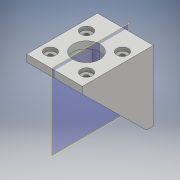
# Autodesk Inventor part: CarroXY-Motor
Saved by Autodesk Inventor 2017 (Build 210142000, 142)
## iProperties
Created: 2020-08-14
Part Number: CarroXY-Motor
Material: Generic
Document SubType Name: Modeling
Designer: ale
Density: 1 g/cm^3
Appearance: Default
Author: ale
Autodesk Inventor part; units mm, degrees
ref_plane "YZ Plane" through (0, 0, 0) normal (1, 0, 0) x (0, 1, 0)
ref_plane "XZ Plane" through (0, 0, 0) normal (0, 1, 0) x (-1, 0, 0)
ref_plane "XY Plane" through (0, 0, 0) normal (0, 0, 1) x (1, 0, 0)
sketch "Sketch1" plane through (0, 0, 0) normal (0, 0, 1) x (1, 0, 0)
  line L0 (-24, 27.5) -> (24, 27.5)
  line L1 (24, 27.5) -> (24, -27.5)
  line L2 (24, -27.5) -> (-24, -27.5)
  line L3 (-24, -27.5) -> (-24, 27.5)
  line L4 (-24, 27.5) -> (24, -27.5) construction
  line L5 (24, 27.5) -> (-24, -27.5) construction
  circle A0 centre (0, 0) radius 11.5
  line L6 (-15.5, 15.5) -> (15.5, -15.5) construction
  line L7 (15.5, 15.5) -> (-15.5, -15.5) construction
  circle A1 centre (-15.5, 15.5) radius 2
  circle A2 centre (15.5, 15.5) radius 2
  circle A3 centre (-15.5, -15.5) radius 2
  circle A4 centre (15.5, -15.5) radius 2
  dimension "d0" = 48
  dimension "d1" = 55
  dimension "d2" = 23
  dimension "d3" = 31
  dimension "d4" = 31
  dimension "d5" = 4
  dimension "d6" = 4
  dimension "d7" = 4
  dimension "d8" = 4
  constraints: 16 end point, 5 centre point, 5 coincident, 4 midpoint, 2 parallel, 1 horizontal, 1 perpendicular
  measures "d0" distance of L1.end L2.end
  measures "d1" distance of L0.end L1.end
  measures "d2" diameter of A0
  measures "d3" distance of L6.end L7.end
  measures "d4" distance of L7.start L6.end
  measures "d5" diameter of A1
  measures "d6" diameter of A2
  measures "d7" diameter of A3
  measures "d8" diameter of A4
extrude "Extrusion1" add sketch "Sketch1" along normal blind 6
sketch "Sketch2" plane through (0, 0, 6) normal (0, 0, 1) x (1, 0, 0)
  circle A0 centre (-15.5, 15.5) radius 2 projected
  circle A1 centre (15.5, 15.5) radius 2 projected
  circle A2 centre (15.5, -15.5) radius 2 projected
  circle A3 centre (-15.5, -15.5) radius 2 projected
  point P0 (0, 0)
  constraints: 4 coincident
hole "Hole1" at (-15.5, 15.5, 6) at (15.5, 15.5, 6) at (15.5, -15.5, 6) at (-15.5, -15.5, 6) direction (0, 0, -1) diameter 4 end through all counterbore diameter 10 counterbore depth 3
sketch "Sketch4" plane through (-24, 27.5, 0) normal (0, 1, 0) x (1, 0, 0)
  line L0 (0, 0) -> (0, -6) projected
  line L1 (0, -6) -> (48, -6)
  line L2 (48, -6) -> (48, 54)
  line L3 (48, 54) -> (0, 54)
  line L4 (0, 54) -> (0, -6)
  point P0 (24, 0)
  dimension "d20" = 60
  constraints: 8 end point, 2 parallel, 1 horizontal, 1 perpendicular
  measures "d20" distance of L2.end L1.end
extrude "Extrusion2" add sketch "Sketch4" along normal blind 6
sketch "Sketch5" plane through (-24, 27.5, 0) normal (0, -1, 0) x (1, 0, 0)
  arc A0 (7.75, -44) -> (12.25, -44) centre (10, -44) ccw
  line L0 (0, -54) -> (0, 0) projected
  line L1 (0, -27) -> (48, -27)
  line L2 (48, 6) -> (48, -54) projected
  line L3 (24, 0) -> (24, -54)
  line L4 (48, -54) -> (0, -54) projected
  arc A1 (12.25, -10) -> (7.75, -10) centre (10, -10) ccw
  line L5 (7.75, -44) -> (7.75, -10)
  line L6 (12.25, -10) -> (12.25, -44)
  arc A2 (35.75, -44) -> (40.25, -44) centre (38, -44) ccw
  arc A3 (40.25, -10) -> (35.75, -10) centre (38, -10) ccw
  line L7 (40.25, -44) -> (40.25, -10)
  line L8 (35.75, -10) -> (35.75, -44)
  dimension "d23" = 4.5
  dimension "d25" = 10
  dimension "d26" = 10
  constraints: 12 end point, 8 point on circle, 7 symmetric about line, 4 centre point, 2 midpoint, 2 tangent, 1 horizontal, 1 parallel, 1 point on line, 3 other
  measures "d23" diameter of A0
  measures "d25" horizontal distance of L0.start A0.centre
  measures "d26" horizontal distance of L0.start A0.centre
extrude "Extrusion3" cut sketch "Sketch5" against normal through all contours L5 L1 L6 A0 | L5 A1 L6 L1 | L8 A3 L7 L1 | L1 L7 A2 L8
sketch "Sketch6" plane through (-24, -27.5, 0) normal (-1, 0, 0) x (0, 0, 1)
  line L0 (6, 0) -> (6, 61) projected
  line L1 (6, 0) -> (0, 0)
  line L2 (-54, 55) -> (0, 55) projected
  line L3 (0, 0) -> (-54, 55)
  line L4 (-54, 55) -> (-54, 61)
  line L5 (-54, 61) -> (6, 61) projected
  line L6 (-54, 61) -> (6, 61)
  line L7 (6, 0) -> (6, 61) projected
  line L8 (6, 61) -> (6, 0)
  line L9 (0, 0) -> (6, 0) projected
  line L10 (6, 0) -> (0, 0)
  point P0 (0, 27.5)
  constraints: 12 end point, 4 perpendicular, 1 horizontal
extrude "Extrusion4" add sketch "Sketch6" against normal blind 2
ref_plane "Work Plane1" through (0, -27.5, 6) normal (-1, 0, 0) x (0, 0, 1)
mirror "Mirror1" about plane through (0, -27.5, 6) normal (-1, 0, 0) of "Extrusion4"
body "Solid1"
